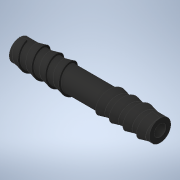
# Autodesk Inventor part: Dribblerschnecke
Saved by Autodesk Inventor 2020 (Build 240168000, 168)
## iProperties
Part Number: Dribblerschnecke
Material: Rubber, Silicone
Document SubType Name: Modeling
Designer: rYan
Mass: 61.7371 g
Surface Area: 150.716 cm^2
Volume: 49.3897 cm^3
Density: 1.25 g/cm^3
Appearance: Gummi - schwarz
Author: rYan
Autodesk Inventor part; units mm, degrees
ref_plane "YZ Plane" through (0, 0, 0) normal (1, 0, 0) x (0, 1, 0)
ref_plane "XZ Plane" through (0, 0, 0) normal (0, 1, 0) x (-1, 0, 0)
ref_plane "XY Plane" through (0, 0, 0) normal (0, 0, 1) x (1, 0, 0)
sketch "Skizze1" plane through (0, 0, 0) normal (1, 0, 0) x (0, 1, 0)
  circle A0 centre (0, 0) radius 3
  circle A1 centre (0, 0) radius 5.5
  dimension "d0" = 6
  dimension "d1" = 11
  constraints: 2 centre point, 2 coincident
  measures "d0" diameter of A0
  measures "d1" diameter of A1
extrude "Extrusion1" add sketch "Skizze1" along normal blind 36
sketch "Skizze3" plane through (0, 0, 0) normal (0, 1, 0) x (-1, 0, 0)
  line L0 (-36, 5.5) -> (-32, 5.5)
  line L1 (-32, 5.5) -> (-32.1763, 6.5)
  line L2 (-32.1763, 6.5) -> (-36, 5.6)
  line L3 (-36, 5.6) -> (-36, 5.5)
  line L4 (-36, 5.5) -> (-36, -5.5) construction
  line L5 (0, -5.5) -> (0, 5.5) construction
  point P0 (0, 0)
  dimension "d16" = 4
  dimension "d17" = 80
  dimension "d18" = 1
  dimension "d19" = 0.1
  constraints: 8 end point, 1 horizontal, 1 vertical
  measures "d16" distance of L0.start L0.end
  measures "d17" angle of L1 L0
  measures "d18" distance from line of L0 L1.end
  measures "d19" distance of L2.end L0.start
coil "Spirale1" sketch "Skizze3" operation add axis through (-10, 0, 0) along (-1, 0, 0) pitch 7 turns 3.5 hand left
mirror "Spiegeln1" about plane through (0, 0, 0) normal (1, 0, 0) of "Extrusion1", "Spirale1"
sketch "Sketch7" plane through (36, 0, 0) normal (1, 0, 0) x (0, 0, -1)
  line L0 (-10, -11) -> (10, -11)
  line L1 (10, -11) -> (10, 11)
  line L2 (10, 11) -> (-10, 11)
  line L3 (-10, 11) -> (-10, -11)
  line L4 (-10, -11) -> (10, 11) construction
  line L5 (10, -11) -> (-10, 11) construction
  point P0 (0, 0)
  constraints: 12 end point, 2 midpoint, 2 parallel, 1 horizontal, 1 perpendicular
extrude "Extrusion5" add sketch "Sketch7" along normal blind 10 and the other way blind 82 separate body
sketch "Sketch8" plane through (-46, 0, 0) normal (-1, 0, 0) x (0, 0, -1)
  circle A0 centre (0, 0) radius 3.5
  dimension "d34" = 7
  constraints: 1 centre point, 1 coincident
  measures "d34" diameter of A0
extrude "Extrusion6" add sketch "Sketch8" against normal up to surface (92 mm away) separate body
body "Solid2"
body "Solid3"
